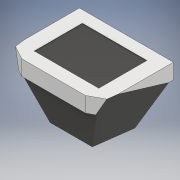
# Autodesk Inventor part: TV
Saved by Autodesk Inventor 2017 (Build 210142000, 142)
## iProperties
Created: 2017-10-02
Part Number: TV
Material: ABS Plastic
Document SubType Name: Modeling
Designer: Felipe
Density: 1.06 g/cm^3
Appearance: Smooth - Black
Author: Felipe
Autodesk Inventor part; units mm, degrees
ref_plane "YZ Plane" through (0, 0, 0) normal (1, 0, 0) x (0, 1, 0)
ref_plane "XZ Plane" through (0, 0, 0) normal (0, 1, 0) x (-1, 0, 0)
ref_plane "XY Plane" through (0, 0, 0) normal (0, 0, 1) x (1, 0, 0)
sketch "Sketch1" plane through (0, 0, 0) normal (0, 0, 1) x (1, 0, 0)
  line L0 (130, 0) -> (670, 0)
  line L1 (800, 70) -> (800, 620)
  line L2 (800, 620) -> (0, 620)
  line L3 (0, 620) -> (0, 70)
  line L4 (0, 70) -> (130, 0)
  line L5 (670, 0) -> (800, 70)
  line L6 (400, 620) -> (400, 0) construction
  point P0 (0, 0)
  dimension "d0" = 800
  dimension "d1" = 620
  dimension "d2" = 550
  dimension "d3" = 550
  dimension "d4" = 270
  dimension "d5" = 270
  dimension "d6" = 70
  dimension "d7" = 70
  dimension "d8" = 130
  dimension "d9" = 130
  constraints: 14 end point, 2 midpoint, 2 parallel, 1 horizontal, 1 perpendicular
  measures "d0" distance of L1.end L2.end
  measures "d1" distance of L2.end point (0, 0)
  measures "d2" distance from line of L1.start L2
  measures "d3" distance from line of L3.end L2
  measures "d4" distance of L0.start L6.end
  measures "d5" distance from line of L0.end L6
  measures "d6" vertical distance of L0.start L3.end
  measures "d7" vertical distance of L1.start L0.end
  measures "d8" horizontal distance of L3.end L0.start
  measures "d9" horizontal distance of L0.end L1.start
extrude "Extrusion1" add sketch "Sketch1" along normal blind 500
sketch "Sketch2" plane through (800, 70, 0) normal (1, 0, 0) x (0, 0, -1)
  line L0 (-370, -31) -> (0, 80)
  line L1 (0, 80) -> (0, -70)
  line L2 (0, -70) -> (-370, -70)
  line L3 (0, 550) -> (-500, 550) projected
  line L4 (-370, 511) -> (0, 400)
  line L5 (0, 400) -> (0, 550)
  line L6 (0, 550) -> (-370, 550)
  line L7 (-370, -31) -> (-370, -70)
  line L8 (0, -70) -> (-500, -70) projected
  line L9 (-370, 511) -> (-370, 550)
  line L10 (-500, -70) -> (-500, 0) projected
  line L11 (-500, 0) -> (-500, 550) projected
  dimension "d12" = 320
  dimension "d15" = 150
  dimension "d16" = 150
  dimension "d17" = 130
  dimension "d18" = 130
  constraints: 16 end point, 4 perpendicular, 4 point on line, 1 coincident
  measures "d12" distance of L0.end L4.end
  measures "d15" distance of L4.end L5.end
  measures "d16" distance of L0.end L1.end
  measures "d17" distance between parallel lines of L10 L7
  measures "d18" distance between parallel lines of L11 L9
extrude "Extrusion2" cut sketch "Sketch2" against normal through all
sketch "Sketch3" plane through (0, 0, 500) normal (0, 0, 1) x (1, 0, 0)
  line L0 (125, 520) -> (675, 520)
  line L1 (675, 520) -> (675, 110)
  line L2 (675, 110) -> (125, 110)
  line L3 (125, 110) -> (125, 520)
  line L4 (800, 620) -> (0, 620) projected
  line L5 (0, 150) -> (0, 470) projected
  line L6 (800, 70) -> (800, 620) projected
  point P0 (0, 0)
  dimension "d21" = 100
  dimension "d22" = 125
  dimension "d23" = 125
  dimension "d24" = 40
  dimension "d33" = 550
  dimension "d34" = 410
  constraints: 8 end point, 2 parallel, 1 horizontal, 1 perpendicular
  measures "d21" distance between parallel lines of L4 L0
  measures "d22" distance between parallel lines of L5 L3
  measures "d23" distance between parallel lines of L6 L1
  measures "d24" distance from line of L6.start L2
  measures "d33" distance of L0.start L0.end
  measures "d34" distance of L2.end L0.start
extrude "Extrusion3" cut sketch "Sketch3" against normal blind 5
sketch "Sketch4" plane through (0, 581, 370) normal (0, 0.9578, -0.2873) x (1, 0, 0)
  line L0 (800, 0) -> (0, 0) projected
  line L1 (800, 0) -> (580, 478.2427)
  line L2 (800, 478.2427) -> (0, 478.2427) projected
  line L3 (0, 0) -> (220, 478.2427)
  line L4 (220, 478.2427) -> (0, 478.2427)
  line L5 (800, -11.2066) -> (0, -11.2066) projected
  line L6 (0, 0) -> (0, 386.2913) projected
  line L7 (0, 478.2427) -> (0, 0)
  line L8 (800, 0) -> (800, 478.2427)
  line L9 (800, 245.8102) -> (800, 22.3174) projected
  line L10 (800, 478.2427) -> (580, 478.2427)
  point P0 (0, 521.3448)
  dimension "d27" = 360
  dimension "d28" = 220
  dimension "d30" = 220
  constraints: 12 end point, 3 collinear, 1 parallel, 1 point on line
  measures "d27" distance of L1.end L3.end
  measures "d28" distance of L2.start L1.end
  measures "d30" distance of L2.end L3.end
extrude "Extrusion4" cut sketch "Sketch4" against normal through all contours L1 L2 L8 | L6 L7 L2 L3
body "Solid1"
